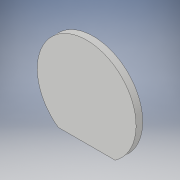
# Autodesk Inventor part: MiddlePiece3
Saved by Autodesk Inventor 2019 (Build 230136000, 136)
## iProperties
Created: 2020-02-13
Part Number: MiddlePiece3
Material: Generic
Document SubType Name: Modeling
Designer: student
Density: 1 g/cm^3
Appearance: Default
Author: student
Autodesk Inventor part; units mm, degrees
ref_plane "YZ Plane" through (0, 0, 0) normal (1, 0, 0) x (0, 1, 0)
ref_plane "XZ Plane" through (0, 0, 0) normal (0, 1, 0) x (-1, 0, 0)
ref_plane "XY Plane" through (0, 0, 0) normal (0, 0, 1) x (1, 0, 0)
sketch "Sketch1" plane through (0, 0, 0) normal (0, 0, 1) x (1, 0, 0)
  circle A0 centre (0, 0) radius 34.925
  dimension "d0" = 69.85
  constraints: 1 centre point, 1 coincident
  measures "d0" diameter of A0
extrude "Extrusion1" add sketch "Sketch1" along normal blind 4.699
sketch "Sketch2" plane through (0, 0, 4.699) normal (0, 0, 1) x (1, 0, 0)
  circle A0 centre (0, 0) radius 34.925 projected
  line L0 (-69.2676, -34.925) -> (88.3759, -34.925) construction
  circle A1 centre (0, 0) radius 34.925 projected
  circle A2 centre (0, 0) radius 34.925 projected
  line L1 (-20.0805, -34.925) -> (20.0805, -34.925)
  line L2 (20.0805, -34.925) -> (20.0805, -28.575)
  line L3 (20.0805, -28.575) -> (-20.0805, -28.575)
  line L4 (-20.0805, -28.575) -> (-20.0805, -34.925)
  dimension "d3" = 6.35
  constraints: 10 end point, 3 horizontal, 2 parallel, 1 perpendicular, 1 point on line, 4 other
  measures "d3" distance of L3.end L1.start
extrude "Extrusion2" cut sketch "Sketch2" against normal through all contours L3 A0 | A0 L1 L4 | L2 L1 A0 picked at (-4.6231, -29.7344)
body "Solid1"
